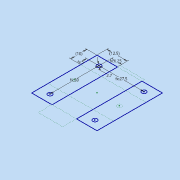
# Autodesk Inventor part: Part7
Saved by Autodesk Inventor 2016 SP1 (Build 200210100, 210)
## iProperties
Created: 2016-03-17
Part Number: Part7
Material: Generic
Document SubType Name: Modeling
Designer: Mohamed A.
Density: 1 g/cm^3
Appearance: Default
Author: Mohamed A.
Autodesk Inventor part; units mm, degrees
ref_plane "YZ Plane" through (0, 0, 0) normal (1, 0, 0) x (0, 1, 0)
ref_plane "XZ Plane" through (0, 0, 0) normal (0, 1, 0) x (-1, 0, 0)
ref_plane "XY Plane" through (0, 0, 0) normal (0, 0, 1) x (1, 0, 0)
sketch "Sketch1" plane through (0, 0, 0) normal (0, 0, 1) x (1, 0, 0)
  circle A0 centre (13.75, 0) radius 1.35 projected
  circle A1 centre (-13.75, 0) radius 1.35 projected
  line L0 (-20, -20) -> (20, -20) construction
  line L1 (20, -20) -> (20, 20) construction
  line L2 (20, 20) -> (-20, 20) construction
  line L3 (-20, 20) -> (-20, -20) construction
  line L4 (7.5, 21.5731) -> (-7.5, 21.5731) construction
  line L5 (-7.5, 21.5731) -> (-7.5, -28.4269) construction
  line L6 (-7.5, -28.4269) -> (7.5, -28.4269) construction
  line L7 (7.5, -28.4269) -> (7.5, 21.5731) construction
  line L8 (20, 20) -> (20, -20)
  line L9 (7.5, -20) -> (20, -20)
  line L10 (7.5, -20) -> (7.5, 20)
  line L11 (7.5, 20) -> (20, 20)
  line L12 (-7.5, 20) -> (-7.5, -20)
  line L13 (-7.5, -20) -> (-20, -20)
  line L14 (-20, -20) -> (-20, 20)
  line L15 (-20, 20) -> (-7.5, 20)
  circle A2 centre (-13.75, 0) radius 1.35 construction
  circle A3 centre (13.75, 0) radius 1.35 construction
  line L16 (20, 10) -> (-20, 10) construction
  line L17 (-20, 10) -> (-20, -10) construction
  line L18 (-20, -10) -> (20, -10) construction
  line L19 (20, -10) -> (20, 10) construction
  circle A4 centre (-13.75, 15) radius 1.35
  circle A5 centre (13.75, 15) radius 1.35
  circle A6 centre (-13.75, -15) radius 1.35
  circle A7 centre (13.75, -15) radius 1.35
  circle A8 centre (-13.75, -15) radius 1.35 projected
  circle A9 centre (13.75, -15) radius 1.35 projected
  circle A10 centre (13.75, 15) radius 1.35 projected
  circle A11 centre (-13.75, 15) radius 1.35 projected
  point P0 (0, 0)
  dimension "d0" = 2.7
  dimension "d1" = 10
  dimension "d2" = 5
  dimension "d3" = 12.5
  dimension "d4" = 6.25
  dimension "d7" = 27.5
  dimension "d10" = 30
  constraints: 16 end point, 8 point on line, 6 collinear, 4 centre point, 1 horizontal, 1 perpendicular, 1 vertical, 6 other
  measures "d0" diameter of A4
  measures "d1" distance between parallel lines of L16 L2
  measures "d2" distance from line of L16 A4.centre
  measures "d3" distance between parallel lines of L14 L12
  measures "d4" distance from line of L12 A4.centre
  measures "d7" distance of A4.centre A5.centre
  measures "d10" distance of A4.centre A6.centre
extrude "Extrusion1" add sketch "Sketch1" along normal blind 3
equation "\"d2\" = 0.5 * d1"
equation "\"d4\" = 0.5 * d3"
body "Solid1"
